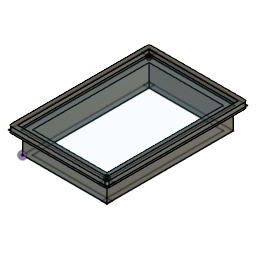
Reservoir_Spacer (Autodesk Fusion 360 design; units mm, degrees)
Autodesk Fusion 360 part; units mm, degrees
sketch "Sketch1" plane through (0, 0, 0) normal (0, 0, 1) x (1, 0, 0)
  line L0 (0, 0) -> (84.5, 0)
  line L1 (84.5, 0) -> (84.5, 126.75)
  line L2 (84.5, 126.75) -> (0, 126.75)
  line L3 (0, 126.75) -> (0, 0)
  line L4 (0, 126.75) -> (5, 126.75)
  line L5 (5, 126.75) -> (5, 121.75)
  line L6 (5, 121.75) -> (0, 121.75)
  line L7 (0, 121.75) -> (0, 126.75)
  line L8 (84.5, 0) -> (79.5, 0)
  line L9 (79.5, 0) -> (79.5, 5)
  line L10 (79.5, 5) -> (84.5, 5)
  line L11 (84.5, 5) -> (84.5, 0)
  line L12 (5, 121.75) -> (79.5, 121.75)
  line L13 (79.5, 121.75) -> (79.5, 5)
  line L14 (79.5, 5) -> (5, 5)
  line L15 (5, 5) -> (5, 121.75)
  dimension "d1" = 84.5
  dimension "d2" = 126.75
  dimension "d3" = 5
  dimension "d4" = 5
  dimension "d5" = 5
  dimension "d6" = 5
  constraint horizontal L0
  constraint vertical L1
  constraint horizontal L2
  constraint vertical L3
  constraint coincident L0.start L3.end
  constraint horizontal L4
  constraint vertical L5
  constraint horizontal L6
  constraint vertical L7
  constraint horizontal L8
  constraint vertical L9
  constraint horizontal L10
  constraint vertical L11
  constraint horizontal L12
  constraint vertical L13
  constraint horizontal L14
  constraint vertical L15
  measures "d1" distance of L0.start L0.end
  measures "d2" distance of L0.start L2.end
  measures "d3" distance of L2.end L4.end
  measures "d4" distance of L2.end L6.end
  measures "d5" distance of L0.end L8.end
  measures "d6" distance of L0.end L10.end
extrude "Extrude1" add sketch "Sketch1" along normal blind 22 contours L0 L3 L6 L9 L14 L15 | L0 L1 L8 L9 L10 L11 | L2 L3 L4 L5 L6 L7 | L1 L2 L5 L10 L12 L13 makes body 1
sketch "Sketch2" plane through (0, 0, 22) normal (0, 0, 1) x (-1, 0, 0)
  line L0 (-79.5, -5) -> (-5, -5)
  line L1 (-5, -5) -> (-5, -121.75)
  line L2 (-5, -121.75) -> (-79.5, -121.75)
  line L3 (-79.5, -121.75) -> (-79.5, -5)
  line L4 (-84.5, -126.75) -> (0, -126.75)
  line L5 (0, -126.75) -> (0, 0)
  line L6 (0, 0) -> (-84.5, 0)
  line L7 (-84.5, 0) -> (-84.5, -126.75)
  line L8 (0, -126.75) -> (7, -126.75)
  line L9 (7, -126.75) -> (7, -133.75)
  line L10 (7, -133.75) -> (0, -133.75)
  line L11 (0, -133.75) -> (0, -126.75)
  line L12 (-84.5, 0) -> (-91.5, 0)
  line L13 (-91.5, 0) -> (-91.5, 7)
  line L14 (-91.5, 7) -> (-84.5, 7)
  line L15 (-84.5, 7) -> (-84.5, 0)
  line L16 (7, -133.75) -> (-91.5, -133.75)
  line L17 (-91.5, -133.75) -> (-91.5, 7)
  line L18 (-91.5, 7) -> (7, 7)
  line L19 (7, 7) -> (7, -133.75)
  line L20 (0, -126.75) -> (0.5, -126.75)
  line L21 (0.5, -126.75) -> (0.5, -127.25)
  line L22 (0.5, -127.25) -> (0, -127.25)
  line L23 (0, -127.25) -> (0, -126.75)
  line L24 (-84.5, 0) -> (-85, 0)
  line L25 (-85, 0) -> (-85, 0.5)
  line L26 (-85, 0.5) -> (-84.5, 0.5)
  line L27 (-84.5, 0.5) -> (-84.5, 0)
  line L28 (0.5, -127.25) -> (-85, -127.25)
  line L29 (-85, -127.25) -> (-85, 0.5)
  line L30 (-85, 0.5) -> (0.5, 0.5)
  line L31 (0.5, 0.5) -> (0.5, -127.25)
  dimension "d9" = 7
  dimension "d10" = 7
  dimension "d11" = 7
  dimension "d12" = 7
  dimension "d24" = 0.5
  dimension "d25" = 0.5
  dimension "d26" = 0.5
  dimension "d27" = 0.5
  constraint horizontal L8
  constraint vertical L9
  constraint horizontal L10
  constraint vertical L11
  constraint coincident L4.end L5.start
  constraint horizontal L12
  constraint vertical L13
  constraint horizontal L14
  constraint vertical L15
  constraint coincident L6.end L7.start
  constraint horizontal L16
  constraint vertical L17
  constraint horizontal L18
  constraint vertical L19
  constraint horizontal L20
  constraint vertical L21
  constraint horizontal L22
  constraint vertical L23
  constraint horizontal L24
  constraint vertical L25
  constraint horizontal L26
  constraint vertical L27
  constraint horizontal L28
  constraint vertical L29
  constraint horizontal L30
  constraint vertical L31
  measures "d9" distance of L4.end L8.end
  measures "d10" distance of L4.end L10.end
  measures "d11" distance of L6.end L12.end
  measures "d12" distance of L6.end L14.end
  measures "d24" distance of L4.end L20.end
  measures "d25" distance of L6.end L24.end
  measures "d26" distance of L6.end L26.end
  measures "d27" distance of L4.end L22.end
extrude "Extrude2" add sketch "Sketch2" along normal blind 4 separate body contours L8 L15 L18 L19 L30 L31 | L8 L9 L10 L11 L16 L19 L21 L22 L28 L31 | L11 L12 L16 L17 L28 L29 | L12 L13 L14 L15 L17 L18 L25 L26 L29 L30 makes body 2
chamfer "Chamfer1" distance 2 angle 45 4 edges at (85, 63.375, 26) (42.25, -0.5, 26) (-0.5, 63.375, 26) (42.25, 127.25, 26) on bodies 2
extrude "Extrude3" add sketch "Sketch2" against normal blind 2 contours L4 L7 L11 L12 L23 L24 L28 L29 | L5 L6 L8 L15 L20 L27 L30 L31 | L8 L11 L20 L21 L22 L23 L28 L31 | L12 L15 L24 L25 L26 L27 L29 L30 | L8 L15 L18 L19 L30 L31 | L8 L9 L10 L11 L16 L19 L21 L22 L28 L31 | L11 L12 L16 L17 L28 L29 | L12 L13 L14 L15 L17 L18 L25 L26 L29 L30 bodies 1 2
fillet "Fillet1" radius 2 4 edges at (-7, -7, 24) (91.5, -7, 24) (-7, 133.75, 24) (91.5, 133.75, 24) on bodies 1 2
